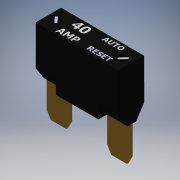
# Autodesk Inventor part: MX5-A40
Saved by Autodesk Inventor 2017.1 (Build 211199000, 199)
## iProperties
Category: Bag #3
Company: Autodesk Inc.
Created: 2016-12-24
Part Number: MX5-A40
Document SubType Name: Modeling
Designer: Autodesk Inc.
Density: 1 g/cm^3
Catalog Web Link: http://www.snapaction.net/pdf/MX5%20Spec%20Sheet.pdf
Description: Circuit breaker 40 amp
Vendor: Snap Action
Material: Generic
Appearance: Glossy - Black
Author: Autodesk Inc.
Keywords: Gray Tote
Autodesk Inventor part; units mm, degrees
note: some values were not read from the file. Chosen so that the rebuilt part matches the saved one: direction of "Emboss1"; direction of "Emboss4".
sketch "Sketch1" plane through (0, 0, 0) normal (0, 0, 1) x (1, 0, 0)
  line L0 (0, 0) -> (28.956, 0)
  line L1 (28.956, 0) -> (28.956, 18.288)
  line L2 (28.956, 18.288) -> (0, 18.288)
  line L3 (0, 18.288) -> (0, 0)
  dimension "d0" = 28.956
  dimension "d1" = 18.288
  constraints: 8 end point, 2 parallel, 1 horizontal, 1 perpendicular
  measures "d0" distance of L1.end L2.end
  measures "d1" distance of L0.end L1.end
extrude "Extrusion1" add sketch "Sketch1" against normal blind 8.89
sketch "Sketch2" plane through (28.956, 0, 0) normal (1, 0, 0) x (0, 0, -1)
  line L0 (0, 0) -> (0, 18.288) projected
  line L1 (0, 0) -> (8.89, 0) projected
  line L2 (2.9633, 0) -> (0, 4.572)
  dimension "d4" = 4.572
  dimension "d5" = 2.9633
  constraints: 2 end point, 2 point on line
  measures "d4" vertical distance of L2.start L2.end
  measures "d5" distance of L2.start L0.start
extrude "Extrusion2" cut sketch "Sketch2" against normal blind 7.112
ref_plane "Work Plane1" through (14.478, 0, -8.89) normal (1, 0, 0) x (0, 0, -1)
mirror "Mirror1" about plane through (14.478, 0, -8.89) normal (1, 0, 0) of "Extrusion2"
ref_plane "Work Plane2" through (0, 0, -4.445) normal (0, 0, 1) x (1, 0, 0)
mirror "Mirror2" about plane through (0, 0, -4.445) normal (0, 0, 1) of "Extrusion2", "Mirror1"
sketch "Sketch4" plane through (21.844, 0, -2.9633) normal (0, -1, 0) x (1, 0, 0)
  line L0 (7.112, 0) -> (7.112, -2.9633) projected
  line L1 (7.112, -1.7728) -> (-0.889, -1.7728)
  line L2 (-0.889, -1.7728) -> (-0.889, -0.96)
  line L3 (-0.889, -0.96) -> (7.112, -0.96)
  line L4 (7.112, -0.96) -> (7.112, -1.7728)
  point P0 (-21.844, 2.9633)
  point P1 (-0.889, -1.3664)
  point P2 (7.112, -1.3664)
  dimension "d13" = 8.001
  dimension "d14" = 0.8128
  constraints: 8 end point, 2 midpoint, 2 parallel, 1 horizontal, 1 horizontal alignment, 1 perpendicular, 1 point on line
  measures "d13" distance of L2.end L3.end
  measures "d14" distance of L1.end L2.end
extrude "Extrusion4" add sketch "Sketch4" along normal blind 12.446
chamfer "Chamfer1" distance 2.54 distance2 1.27 1 edges at (20.955, -12.446, -4.3297) measured on face at (20.955, -4.1487, -4.1942)
chamfer "Chamfer2" distance 2.54 distance2 1.27 1 edges at (28.956, -12.446, -4.3297) measured on face at (28.956, 13.716, -5.9267)
chamfer "Chamfer3" distance 2.54 distance2 0.127 1 edges at (24.9555, -12.446, -3.9233) measured on face at (23.622, -6.604, -3.9233)
chamfer "Chamfer4" distance 2.54 distance2 0.127 1 edges at (24.9555, -12.446, -4.7361) measured on face at (26.289, -6.604, -4.7361)
ref_plane "Work Plane3" through (21.844, 0, -2.9633) normal (0, -1, 0) x (1, 0, 0)
mirror "Mirror3" about plane through (14.478, 0, -8.89) normal (1, 0, 0) of "Extrusion4", "Chamfer3", "Chamfer4"
chamfer "Chamfer5" distance 1.27 distance2 2.54 1 edges at (8.001, -12.446, -4.3297) measured on face at (2.667, -12.446, -4.2366)
chamfer "Chamfer6" distance 1.27 distance2 2.54 1 edges at (0, -12.446, -4.3297) measured on face at (2.2437, -12.446, -4.2366)
split_face "Split1"
sketch "Sketch5" plane through (0, 18.288, 0) normal (0, 1, 0) x (1, 0, 0)
  circle A0 centre (26.0604, 4.3297) radius 1.5875
  circle A1 centre (2.8956, 4.3297) radius 1.5875
  line L0 (28.956, 3.9233) -> (28.956, 4.7361) projected
  line L1 (28.956, 8.89) -> (0, 8.89) projected
  line L2 (0, 0) -> (0, 8.89) projected
  line L3 (28.956, 0) -> (0, 0) projected
  line L4 (14.478, 8.89) -> (14.478, 0) construction
  point P0 (28.956, 4.3297)
  dimension "d36" = 3.175
  dimension "d58" = 11.5824
  dimension "d59" = 11.5824
  constraints: 3 midpoint, 2 centre point, 2 end point, 2 horizontal alignment, 1 equal radius, 1 parallel
  measures "d36" diameter of A0
  measures "d58" distance from line of A1.centre L4
  measures "d59" distance from line of L4 A0.centre
extrude "Extrusion5" cut sketch "Sketch5" against normal blind 0.635
ref_plane "Work Plane4" through (0, 23.0505, 0) normal (0, 1, 0) x (1, 0, 0)
sketch "Sketch6" plane through (0, 23.0505, 0) normal (0, 1, 0) x (1, 0, 0)
  line L0 (28.956, 8.89) -> (0, 8.89) projected
  line L1 (5.9022, 7.8551) -> (13.3635, 7.8551) construction
  line L2 (13.3635, 7.8551) -> (13.3635, 1.0349) construction
  line L3 (13.3635, 1.0349) -> (5.9022, 1.0349) construction
  line L4 (5.9022, 1.0349) -> (5.9022, 7.8551) construction
  line L5 (0, 0) -> (0, 8.89) projected
  line L6 (9.5489, 5.4567) -> (9.1364, 5.4567)
  line L7 (9.1364, 5.4567) -> (9.1364, 4.7379)
  line L8 (9.1364, 4.7379) -> (8.3978, 4.7379)
  line L9 (8.3978, 4.7379) -> (8.3978, 5.4567)
  line L10 (8.3978, 5.4567) -> (7.0541, 5.4567)
  line L11 (7.0541, 5.4567) -> (7.0541, 6.0248)
  line L12 (7.0541, 6.0248) -> (8.3731, 7.7933)
  line L13 (8.3731, 7.7933) -> (9.1364, 7.7933)
  line L14 (9.1364, 7.7933) -> (9.1364, 6.005)
  line L15 (9.1364, 6.005) -> (9.5489, 6.005)
  line L16 (9.5489, 6.005) -> (9.5489, 5.4567)
  line L17 (8.3978, 6.005) -> (8.3978, 7.0424)
  line L18 (8.3978, 7.0424) -> (7.6247, 6.005)
  line L19 (7.6247, 6.005) -> (8.3978, 6.005)
  spline S0 degree 2 poles (12.1424, 6.2693) (12.1424, 5.8741) (12.0164, 5.2813) (11.8756, 5.0812) knots 0 0 0 1 2 2 2
  spline S1 degree 2 poles (11.8756, 5.0812) (11.7373, 4.8836) (11.2902, 4.6811) (10.9691, 4.6811) knots 0 0 0 1 2 2 2
  spline S2 degree 2 poles (10.9691, 4.6811) (10.6455, 4.6811) (10.2009, 4.8836) (10.0602, 5.0862) knots 0 0 0 1 2 2 2
  spline S3 degree 2 poles (10.0602, 5.0862) (9.9194, 5.2862) (9.7934, 5.8741) (9.7934, 6.2693) knots 0 0 0 1 2 2 2
  spline S4 degree 2 poles (9.7934, 6.2693) (9.7934, 6.6744) (9.9194, 7.2474) (10.0626, 7.4549) knots 0 0 0 1 2 2 2
  spline S5 degree 2 poles (10.0626, 7.4549) (10.2059, 7.6575) (10.6579, 7.8551) (10.9691, 7.8551) knots 0 0 0 1 2 2 2
  spline S6 degree 2 poles (10.9691, 7.8551) (11.2976, 7.8551) (11.7373, 7.6476) (11.8781, 7.4426) knots 0 0 0 1 2 2 2
  spline S7 degree 2 poles (11.8781, 7.4426) (12.0164, 7.2425) (12.1424, 6.6522) (12.1424, 6.2693) knots 0 0 0 1 2 2 2
  spline S8 degree 2 poles (11.3742, 6.2693) (11.3742, 6.8349) (11.1889, 7.2919) (10.9691, 7.2919) knots 0 0 0 1 2 2 2
  spline S9 degree 2 poles (10.9691, 7.2919) (10.7493, 7.2919) (10.5616, 6.8349) (10.5616, 6.2668) knots 0 0 0 1 2 2 2
  spline S10 degree 2 poles (10.5616, 6.2668) (10.5616, 5.7086) (10.7493, 5.2443) (10.9691, 5.2443) knots 0 0 0 1 2 2 2
  spline S11 degree 2 poles (10.9691, 5.2443) (11.1865, 5.2443) (11.3742, 5.7086) (11.3742, 6.2693) knots 0 0 0 1 2 2 2
  line L20 (6.1103, 0.6874) -> (6.8828, 2.9734)
  line L21 (6.8828, 2.9734) -> (7.5089, 2.9734)
  line L22 (7.5089, 2.9734) -> (8.2814, 0.6874)
  line L23 (8.2814, 0.6874) -> (7.6905, 0.6874)
  line L24 (7.6905, 0.6874) -> (7.5478, 1.1543)
  line L25 (7.5478, 1.1543) -> (6.8291, 1.1543)
  line L26 (6.8291, 1.1543) -> (6.6846, 0.6874)
  line L27 (6.6846, 0.6874) -> (6.1103, 0.6874)
  line L28 (7.4219, 1.5692) -> (7.1885, 2.325)
  line L29 (7.1885, 2.325) -> (6.9532, 1.5692)
  line L30 (6.9532, 1.5692) -> (7.4219, 1.5692)
  line L31 (10.8435, 0.6874) -> (10.2729, 0.6874)
  line L32 (10.2729, 0.6874) -> (10.2729, 2.2028)
  line L33 (10.2729, 2.2028) -> (9.8579, 1.2247)
  line L34 (9.8579, 1.2247) -> (9.4652, 1.2247)
  line L35 (9.4652, 1.2247) -> (9.0502, 2.2028)
  line L36 (9.0502, 2.2028) -> (9.0502, 0.6874)
  line L37 (9.0502, 0.6874) -> (8.5093, 0.6874)
  line L38 (8.5093, 0.6874) -> (8.5093, 2.9734)
  line L39 (8.5093, 2.9734) -> (9.1706, 2.9734)
  line L40 (9.1706, 2.9734) -> (9.6782, 1.8452)
  line L41 (9.6782, 1.8452) -> (10.1821, 2.9734)
  line L42 (10.1821, 2.9734) -> (10.8435, 2.9734)
  line L43 (10.8435, 2.9734) -> (10.8435, 0.6874)
  spline S12 degree 2 poles (13.0757, 2.2528) (13.0757, 2.0935) (12.9738, 1.8045) (12.8794, 1.7082) knots 0 0 0 1 2 2 2
  spline S13 degree 2 poles (12.8794, 1.7082) (12.8219, 1.647) (12.6811, 1.547) (12.5978, 1.5118) knots 0 0 0 1 2 2 2
  spline S14 degree 2 poles (12.5978, 1.5118) (12.5126, 1.4766) (12.3144, 1.4358) (12.1921, 1.4358) knots 0 0 0 1 2 2 2
  line L44 (12.1921, 1.4358) -> (11.892, 1.4358)
  line L45 (11.892, 1.4358) -> (11.892, 0.6874)
  line L46 (11.892, 0.6874) -> (11.3177, 0.6874)
  line L47 (11.3177, 0.6874) -> (11.3177, 2.9734)
  line L48 (11.3177, 2.9734) -> (12.2051, 2.9734)
  spline S15 degree 2 poles (12.2051, 2.9734) (12.4014, 2.9734) (12.6886, 2.9012) (12.8053, 2.8234) knots 0 0 0 1 2 2 2
  spline S16 degree 2 poles (12.8053, 2.8234) (12.9349, 2.7363) (13.0757, 2.451) (13.0757, 2.2528) knots 0 0 0 1 2 2 2
  spline S17 degree 2 poles (12.4866, 2.238) (12.4866, 2.3362) (12.394, 2.4751) (12.331, 2.501) knots 0 0 0 1 2 2 2
  spline S18 degree 2 poles (12.331, 2.501) (12.2495, 2.5362) (12.1013, 2.5473) (11.9735, 2.5473) knots 0 0 0 1 2 2 2
  line L49 (11.9735, 2.5473) -> (11.892, 2.5473)
  line L50 (11.892, 2.5473) -> (11.892, 1.8619)
  line L51 (11.892, 1.8619) -> (11.9327, 1.8619)
  spline S19 degree 2 poles (11.9327, 1.8619) (12.0124, 1.8619) (12.1569, 1.8656) (12.2106, 1.8749) knots 0 0 0 1 2 2 2
  spline S20 degree 2 poles (12.2106, 1.8749) (12.2569, 1.8823) (12.3588, 1.9268) (12.3866, 1.9545) knots 0 0 0 1 2 2 2
  spline S21 degree 2 poles (12.3866, 1.9545) (12.4459, 2.0101) (12.4866, 2.1342) (12.4866, 2.238) knots 0 0 0 1 2 2 2
  point P0 (9.6328, 7.8551)
  point P1 (14.478, 8.89)
  point P2 (5.9022, 4.445)
  point P3 (0, 4.445)
  constraints: 4 midpoint, 1 horizontal, 1 horizontal alignment, 2 other
emboss "Emboss1" sketch "Sketch6" operation cut depth 0.0254 direction (0, -1, 0)
fillet "Fillet1" radius 0.254 8 edges at (0, 11.43, 0) (28.956, 11.43, 0) (28.956, 11.43, -8.89) (0, 11.43, -8.89) (0, 18.288, -4.445) (14.478, 18.288, 0) (14.478, 18.288, -8.89) (28.956, 18.288, -4.445)
ref_plane "Work Plane5" through (0.254, 21.463, -8.636) normal (0, 1, 0) x (1, 0, 0)
sketch "Sketch9" plane through (0.254, 21.463, -8.636) normal (0, 1, 0) x (1, 0, 0)
  line L0 (16.4321, -0.6968) -> (29.8566, -0.6968) construction
  line L1 (29.8566, -0.6968) -> (29.8566, -7.9158) construction
  line L2 (29.8566, -7.9158) -> (16.4321, -7.9158) construction
  line L3 (16.4321, -7.9158) -> (16.4321, -0.6968) construction
  line L4 (27.432, -4.5857) -> (27.432, -4.0269) projected
  line L5 (16.4249, -2.5123) -> (17.0257, -0.7343)
  line L6 (17.0257, -0.7343) -> (17.5127, -0.7343)
  line L7 (17.5127, -0.7343) -> (18.1135, -2.5123)
  line L8 (18.1135, -2.5123) -> (17.6539, -2.5123)
  line L9 (17.6539, -2.5123) -> (17.543, -2.1492)
  line L10 (17.543, -2.1492) -> (16.9839, -2.1492)
  line L11 (16.9839, -2.1492) -> (16.8715, -2.5123)
  line L12 (16.8715, -2.5123) -> (16.4249, -2.5123)
  line L13 (17.445, -1.8264) -> (17.2634, -1.2386)
  line L14 (17.2634, -1.2386) -> (17.0804, -1.8264)
  line L15 (17.0804, -1.8264) -> (17.445, -1.8264)
  spline S0 degree 2 poles (19.0097, -2.5497) (18.651, -2.5497) (18.2648, -2.2039) (18.2648, -1.8697) knots 0 0 0 1 2 2 2
  line L16 (18.2648, -1.8697) -> (18.2648, -0.7343)
  line L17 (18.2648, -0.7343) -> (18.7115, -0.7343)
  line L18 (18.7115, -0.7343) -> (18.7115, -1.8437)
  spline S1 degree 2 poles (18.7115, -1.8437) (18.7115, -2.0296) (18.8512, -2.2111) (19.0097, -2.2111) knots 0 0 0 1 2 2 2
  spline S2 degree 2 poles (19.0097, -2.2111) (19.1639, -2.2111) (19.308, -2.0368) (19.308, -1.8437) knots 0 0 0 1 2 2 2
  line L19 (19.308, -1.8437) -> (19.308, -0.7343)
  line L20 (19.308, -0.7343) -> (19.7546, -0.7343)
  line L21 (19.7546, -0.7343) -> (19.7546, -1.8682)
  spline S3 degree 2 poles (19.7546, -1.8682) (19.7546, -2.1967) (19.3786, -2.5497) (19.0097, -2.5497) knots 0 0 0 1 2 2 2
  line L22 (20.439, -2.5123) -> (20.439, -1.0729)
  line L23 (20.439, -1.0729) -> (19.9131, -1.0729)
  line L24 (19.9131, -1.0729) -> (19.9131, -0.7343)
  line L25 (19.9131, -0.7343) -> (21.4116, -0.7343)
  line L26 (21.4116, -0.7343) -> (21.4116, -1.0729)
  line L27 (21.4116, -1.0729) -> (20.8857, -1.0729)
  line L28 (20.8857, -1.0729) -> (20.8857, -2.5123)
  line L29 (20.8857, -2.5123) -> (20.439, -2.5123)
  spline S4 degree 2 poles (23.2127, -1.6233) (23.2127, -2.0555) (22.7516, -2.5497) (22.351, -2.5497) knots 0 0 0 1 2 2 2
  spline S5 degree 2 poles (22.351, -2.5497) (21.9491, -2.5497) (21.4909, -2.0498) (21.4909, -1.6233) knots 0 0 0 1 2 2 2
  spline S6 degree 2 poles (21.4909, -1.6233) (21.4909, -1.1953) (21.9491, -0.6968) (22.351, -0.6968) knots 0 0 0 1 2 2 2
  spline S7 degree 2 poles (22.351, -0.6968) (22.7516, -0.6968) (23.2127, -1.1925) (23.2127, -1.6233) knots 0 0 0 1 2 2 2
  spline S8 degree 2 poles (22.7516, -1.6233) (22.7516, -1.4633) (22.6868, -1.24) (22.6306, -1.1694) knots 0 0 0 1 2 2 2
  spline S9 degree 2 poles (22.6306, -1.1694) (22.5744, -1.0959) (22.4303, -1.0325) (22.3525, -1.0325) knots 0 0 0 1 2 2 2
  spline S10 degree 2 poles (22.3525, -1.0325) (22.2704, -1.0325) (22.1364, -1.0916) (22.0744, -1.1665) knots 0 0 0 1 2 2 2
  spline S11 degree 2 poles (22.0744, -1.1665) (22.0197, -1.2357) (21.9519, -1.4648) (21.9519, -1.6233) knots 0 0 0 1 2 2 2
  spline S12 degree 2 poles (21.9519, -1.6233) (21.9519, -1.7875) (22.0168, -2.0037) (22.073, -2.0771) knots 0 0 0 1 2 2 2
  spline S13 degree 2 poles (22.073, -2.0771) (22.1292, -2.1506) (22.2747, -2.214) (22.3525, -2.214) knots 0 0 0 1 2 2 2
  spline S14 degree 2 poles (22.3525, -2.214) (22.4317, -2.214) (22.5787, -2.1463) (22.632, -2.0743) knots 0 0 0 1 2 2 2
  spline S15 degree 2 poles (22.632, -2.0743) (22.6896, -1.9964) (22.7516, -1.7904) (22.7516, -1.6233) knots 0 0 0 1 2 2 2
  line L30 (18.2591, -7.9051) -> (17.7159, -7.9051)
  line L31 (17.7159, -7.9051) -> (17.2216, -7.2524)
  line L32 (17.2216, -7.2524) -> (17.0603, -7.2524)
  line L33 (17.0603, -7.2524) -> (17.0603, -7.9051)
  line L34 (17.0603, -7.9051) -> (16.6165, -7.9051)
  line L35 (16.6165, -7.9051) -> (16.6165, -6.1271)
  line L36 (16.6165, -6.1271) -> (17.3312, -6.1271)
  spline S16 degree 2 poles (17.3312, -6.1271) (17.4796, -6.1271) (17.6986, -6.1646) (17.7922, -6.2222) knots 0 0 0 1 2 2 2
  spline S17 degree 2 poles (17.7922, -6.2222) (17.8873, -6.2828) (17.9997, -6.4715) (17.9997, -6.6156) knots 0 0 0 1 2 2 2
  spline S18 degree 2 poles (17.9997, -6.6156) (17.9997, -6.8187) (17.8153, -7.0738) (17.6611, -7.1487) knots 0 0 0 1 2 2 2
  line L37 (17.6611, -7.1487) -> (18.2591, -7.9051)
  spline S19 degree 2 poles (17.5415, -6.6718) (17.5415, -6.6041) (17.4896, -6.5075) (17.4306, -6.4816) knots 0 0 0 1 2 2 2
  spline S20 degree 2 poles (17.4306, -6.4816) (17.3888, -6.4643) (17.2865, -6.4542) (17.2101, -6.4542) knots 0 0 0 1 2 2 2
  line L38 (17.2101, -6.4542) -> (17.0603, -6.4542)
  line L39 (17.0603, -6.4542) -> (17.0603, -6.9326)
  line L40 (17.0603, -6.9326) -> (17.1885, -6.9326)
  spline S21 degree 2 poles (17.1885, -6.9326) (17.2807, -6.9326) (17.4118, -6.9095) (17.4565, -6.8735) knots 0 0 0 1 2 2 2
  spline S22 degree 2 poles (17.4565, -6.8735) (17.4997, -6.8389) (17.5415, -6.7467) (17.5415, -6.6718) knots 0 0 0 1 2 2 2
  line L41 (18.3916, -7.9051) -> (18.3916, -6.1271)
  line L42 (18.3916, -6.1271) -> (19.5933, -6.1271)
  line L43 (19.5933, -6.1271) -> (19.5933, -6.4657)
  line L44 (19.5933, -6.4657) -> (18.8354, -6.4657)
  line L45 (18.8354, -6.4657) -> (18.8354, -6.7784)
  line L46 (18.8354, -6.7784) -> (19.5342, -6.7784)
  line L47 (19.5342, -6.7784) -> (19.5342, -7.117)
  line L48 (19.5342, -7.117) -> (18.8354, -7.117)
  line L49 (18.8354, -7.117) -> (18.8354, -7.5665)
  line L50 (18.8354, -7.5665) -> (19.5933, -7.5665)
  line L51 (19.5933, -7.5665) -> (19.5933, -7.9051)
  line L52 (19.5933, -7.9051) -> (18.3916, -7.9051)
  spline S23 degree 2 poles (20.4448, -7.9368) (20.2402, -7.9368) (19.9319, -7.8576) (19.7993, -7.8) knots 0 0 0 1 2 2 2
  line L53 (19.7993, -7.8) -> (19.7993, -7.3764)
  line L54 (19.7993, -7.3764) -> (19.8397, -7.3764)
  spline S24 degree 2 poles (19.8397, -7.3764) (19.9737, -7.4902) (20.295, -7.6126) (20.4463, -7.6126) knots 0 0 0 1 2 2 2
  spline S25 degree 2 poles (20.4463, -7.6126) (20.4852, -7.6126) (20.6105, -7.5954) (20.648, -7.5781) knots 0 0 0 1 2 2 2
  spline S26 degree 2 poles (20.648, -7.5781) (20.6941, -7.5579) (20.7589, -7.4844) (20.7589, -7.4253) knots 0 0 0 1 2 2 2
  spline S27 degree 2 poles (20.7589, -7.4253) (20.7589, -7.3576) (20.6537, -7.2741) (20.5817, -7.2553) knots 0 0 0 1 2 2 2
  spline S28 degree 2 poles (20.5817, -7.2553) (20.4909, -7.2308) (20.2849, -7.189) (20.1941, -7.1573) knots 0 0 0 1 2 2 2
  spline S29 degree 2 poles (20.1941, -7.1573) (19.9881, -7.0853) (19.8094, -6.8389) (19.8094, -6.6545) knots 0 0 0 1 2 2 2
  spline S30 degree 2 poles (19.8094, -6.6545) (19.8094, -6.4052) (20.2316, -6.0954) (20.5486, -6.0954) knots 0 0 0 1 2 2 2
  spline S31 degree 2 poles (20.5486, -6.0954) (20.707, -6.0954) (21.0211, -6.1603) (21.1451, -6.215) knots 0 0 0 1 2 2 2
  line L55 (21.1451, -6.215) -> (21.1451, -6.6213)
  line L56 (21.1451, -6.6213) -> (21.1062, -6.6213)
  spline S32 degree 2 poles (21.1062, -6.6213) (21.0067, -6.5363) (20.7215, -6.4196) (20.5716, -6.4196) knots 0 0 0 1 2 2 2
  spline S33 degree 2 poles (20.5716, -6.4196) (20.5125, -6.4196) (20.4203, -6.4369) (20.3684, -6.46) knots 0 0 0 1 2 2 2
  spline S34 degree 2 poles (20.3684, -6.46) (20.3267, -6.4787) (20.2661, -6.5536) (20.2661, -6.5997) knots 0 0 0 1 2 2 2
  spline S35 degree 2 poles (20.2661, -6.5997) (20.2661, -6.6689) (20.3627, -6.7481) (20.501, -6.7798) knots 0 0 0 1 2 2 2
  spline S36 degree 2 poles (20.501, -6.7798) (20.5903, -6.8) (20.756, -6.8389) (20.8511, -6.8721) knots 0 0 0 1 2 2 2
  spline S37 degree 2 poles (20.8511, -6.8721) (21.0356, -6.9398) (21.2157, -7.1645) (21.2157, -7.349) knots 0 0 0 1 2 2 2
  spline S38 degree 2 poles (21.2157, -7.349) (21.2157, -7.6141) (20.7993, -7.9368) (20.4448, -7.9368) knots 0 0 0 1 2 2 2
  line L57 (21.4448, -7.9051) -> (21.4448, -6.1271)
  line L58 (21.4448, -6.1271) -> (22.6464, -6.1271)
  line L59 (22.6464, -6.1271) -> (22.6464, -6.4657)
  line L60 (22.6464, -6.4657) -> (21.8885, -6.4657)
  line L61 (21.8885, -6.4657) -> (21.8885, -6.7784)
  line L62 (21.8885, -6.7784) -> (22.5873, -6.7784)
  line L63 (22.5873, -6.7784) -> (22.5873, -7.117)
  line L64 (22.5873, -7.117) -> (21.8885, -7.117)
  line L65 (21.8885, -7.117) -> (21.8885, -7.5665)
  line L66 (21.8885, -7.5665) -> (22.6464, -7.5665)
  line L67 (22.6464, -7.5665) -> (22.6464, -7.9051)
  line L68 (22.6464, -7.9051) -> (21.4448, -7.9051)
  line L69 (23.2905, -7.9051) -> (23.2905, -6.4657)
  line L70 (23.2905, -6.4657) -> (22.7646, -6.4657)
  line L71 (22.7646, -6.4657) -> (22.7646, -6.1271)
  line L72 (22.7646, -6.1271) -> (24.263, -6.1271)
  line L73 (24.263, -6.1271) -> (24.263, -6.4657)
  line L74 (24.263, -6.4657) -> (23.7371, -6.4657)
  line L75 (23.7371, -6.4657) -> (23.7371, -7.9051)
  line L76 (23.7371, -7.9051) -> (23.2905, -7.9051)
  point P0 (-0.254, -8.636)
  point P1 (29.8566, -4.3063)
  point P2 (27.432, -4.3063)
  constraints: 2 midpoint, 1 horizontal alignment, 2 other
emboss "Emboss4" sketch "Sketch9" operation cut depth 0.0025 direction (0, -1, 0)
sketch "Sketch10" plane through (0.254, 18.288, -8.636) normal (0, 1, 0) x (1, 0, 0)
  circle A0 centre (2.6416, -4.3063) radius 1.5875 projected
  line L0 (3.2205, -5.5479) -> (1.4668, -3.6016)
  line L1 (2.6416, -4.3063) -> (2.3436, -4.5748) construction
  line L2 (3.7943, -5.0465) -> (2.0252, -3.0829)
  circle A1 centre (2.6416, -4.3063) radius 1.3699
  point P0 (-0.254, -8.636)
  point P1 (3.3718, -5.7159)
  point P2 (1.3155, -3.4336)
  point P3 (3.9446, -5.2132)
  point P4 (1.8749, -2.9162)
  dimension "d53" = 0.762
  constraints: 8 point on circle, 6 end point, 1 centre point, 1 midpoint, 1 parallel, 1 perpendicular, 1 point on line
  measures "d53" distance between parallel lines of L2 L0
extrude "Extrusion7" add sketch "Sketch10" against normal up to next contours L0 A1 L2
mirror "Mirror4" about plane through (14.478, 0, -8.89) normal (1, 0, 0) of "Extrusion7"
equation "\"d59\" = d58"
body "Solid1"
